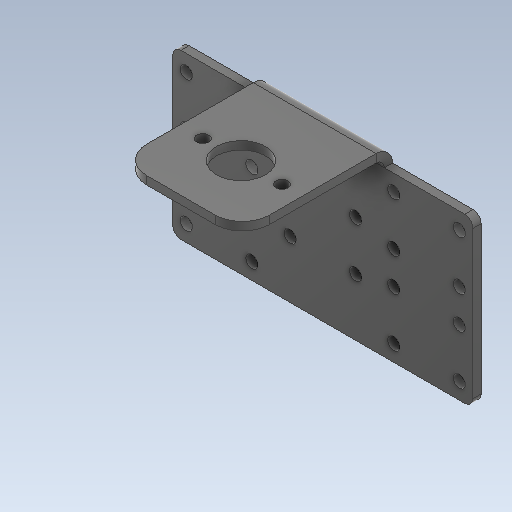
# Autodesk Inventor part: De truc Z chan sat
Saved by Autodesk Inventor 2020 (Build 240168000, 168)
## iProperties
Created: 2021-05-25
Part Number: De truc Z chan sat
Material: Generic
Document SubType Name: Sheet Metal
Designer: admin
Density: 1 g/cm^3
Sheet Metal Rule: Default_mm
Appearance: Smooth - Black
Author: admin
Autodesk Inventor part; units mm, degrees
ref_plane "YZ Plane" through (0, 0, 0) normal (1, 0, 0) x (0, 1, 0)
ref_plane "XZ Plane" through (0, 0, 0) normal (0, 1, 0) x (-1, 0, 0)
ref_plane "XY Plane" through (0, 0, 0) normal (0, 0, 1) x (1, 0, 0)
sketch "Sketch1" plane through (0, 0, 0) normal (0, 0, 1) x (1, 0, 0)
  line L0 (-55, -30) -> (55, -30)
  line L1 (55, -30) -> (55, 30)
  line L2 (55, 30) -> (-55, 30)
  line L3 (-55, 30) -> (-55, -30)
  line L4 (-55, -30) -> (55, 30) construction
  line L5 (55, -30) -> (-55, 30) construction
  line L6 (0, -42) -> (0, 42)
  point P0 (0, 0)
  dimension "d1" = 110
  dimension "d2" = 60
  dimension "d60" = 0
  measures "d1" distance of L2.end L1.end
  measures "d2" distance of L1.end L0.end
  measures "d60" distance from line of point (0, 0) L6
extrude "Plate1" add sketch "Sketch1" along normal blind 3
sketch "Sketch2" plane through (0, 0, 3) normal (0, 0, 1) x (1, 0, 0)
  line L0 (26, -24) -> (50, -24)
  line L1 (50, -24) -> (50, -6)
  line L2 (50, -6) -> (26, -6)
  line L3 (26, -6) -> (26, -24)
  line L4 (26, -24) -> (50, -6) construction
  line L5 (50, -24) -> (26, -6) construction
  circle A0 centre (50, -6) radius 2.25
  circle A1 centre (50, -24) radius 2.25
  circle A2 centre (26, -24) radius 2.25
  circle A3 centre (26, -6) radius 2.25
  line L6 (55, 30) -> (55, -30) projected
  line L7 (55, -30) -> (-55, -30) projected
  point P0 (0, 0)
  point P1 (0, 0)
  point P2 (38, -15)
  dimension "d4" = 24
  dimension "d5" = 18
  dimension "d8" = 4.5
  dimension "d9" = 4.5
  dimension "d10" = 4.5
  dimension "d11" = 4.5
  dimension "d12" = 5
  dimension "d13" = 15
  constraints: 12 end point, 4 centre point, 4 coincident, 2 midpoint, 2 parallel, 1 horizontal, 1 perpendicular
  measures "d4" distance of L2.end L1.end
  measures "d5" distance of L1.end L1.start
  measures "d8" diameter of A0
  measures "d9" diameter of A1
  measures "d10" diameter of A2
  measures "d11" diameter of A3
  measures "d12" distance between parallel lines of L6 L1
  measures "d13" distance from line of L7 point (38, -15)
extrude "Cut1" cut sketch "Sketch2" against normal blind 3 contours L3 A2 L0 | L0 A2 L3 | A1 L1 L0 | L0 L1 A1 | A3 L2 L3 | L3 L2 A3 | A0 L2 L1 | L1 L2 A0
pattern_linear "Rectangular Pattern1" count 2 spacing 30 along (0, 1, 0) of "Cut1"
mirror "Mirror1" about plane through (0, 0, 0) normal (1, 0, 0) of "Cut1", "Rectangular Pattern1"
sketch "Sketch3" plane through (0, 0, 3) normal (0, 0, 1) x (1, 0, 0)
  line L0 (-12, -9) -> (12, -9)
  line L1 (12, -9) -> (12, 9)
  line L2 (12, 9) -> (-12, 9)
  line L3 (-12, 9) -> (-12, -9)
  line L4 (-12, -9) -> (12, 9) construction
  line L5 (12, -9) -> (-12, 9) construction
  circle A0 centre (-12, 9) radius 2.25
  circle A1 centre (12, 9) radius 2.25
  circle A2 centre (12, -9) radius 2.25
  circle A3 centre (-12, -9) radius 2.25
  line L6 (-77, 0) -> (77, 0) projected
  line L7 (0, -42) -> (0, 42) projected
  point P0 (0, 0)
  dimension "d20" = 24
  dimension "d21" = 18
  dimension "d22" = 4.5
  dimension "d23" = 4.5
  dimension "d24" = 4.5
  dimension "d25" = 4.5
  dimension "d26" = 12
  dimension "d27" = 9
  constraints: 12 end point, 4 centre point, 4 coincident, 2 midpoint, 2 parallel, 1 horizontal, 1 perpendicular
  measures "d20" distance of L2.end L1.end
  measures "d21" distance of L1.end L0.end
  measures "d22" diameter of A0
  measures "d23" diameter of A1
  measures "d24" diameter of A2
  measures "d25" diameter of A3
  measures "d26" distance between parallel lines of L7 L1
  measures "d27" distance between parallel lines of L6 L2
extrude "Cut2" cut sketch "Sketch3" against normal blind 3 contours L3 A3 L0 | L0 A3 L3 | A2 L1 L0 | L0 L1 A2 | A0 L2 L3 | L3 L2 A0 | A1 L2 L1 | L1 L2 A1
sketch "Sketch4" plane through (0, 0, 3) normal (0, 0, 1) x (1, 0, 0)
  line L0 (-55, 30) -> (55, 30)
  line L1 (-22.5, 30) -> (22.5, 30)
  line L2 (22.5, 30) -> (22.5, 33)
  line L3 (22.5, 33) -> (-22.5, 33)
  line L4 (-22.5, 33) -> (-22.5, 30)
  point P0 (0, 0)
  point P1 (-50, 30)
  point P2 (50, 30)
  dimension "d30" = 45
  dimension "d31" = 3
  dimension "d32" = 22.5
  measures "d30" distance of L3.end L2.end
  measures "d31" distance of L2.end L1.end
  measures "d32" distance from line of L4 point (0, 0)
sheet face with bend "Face2" sketch "Sketch4" thickness 3 toward (0, 0, -1) bend radius 3
bend "Bend1"
sketch "Sketch5" plane through (-22.5, 33, 3) normal (0, 1, 0) x (-1, 0, 0)
  line L0 (-45, 0) -> (0, 0)
  line L1 (0, 0) -> (0, 52)
  line L2 (0, 52) -> (-45, 52)
  line L3 (-45, 52) -> (-45, 0)
  constraints: 6 end point, 1 horizontal, 1 perpendicular, 1 vertical
edge flange "Flange1" height 55 angle 90 thickness 3 bend radius 3 thickness toward (0, 1, 0) relief tear relief width 3 relief depth 1.5 edges at (0, 33, 3) wall of the first edge with corners at (22.5, 33, 3) (-22.5, 33, 3) (-22.5, 33, 55) (22.5, 33, 55)
bend "Bend2"
corner "Corner1"
sketch "Sketch6" plane through (-22.5, 36, 55) normal (0, 1, 0) x (1, 0, 0)
  circle A0 centre (22.5, 22) radius 9
  line L0 (0, 55) -> (45, 55) projected
  circle A1 centre (37.5, 22) radius 2.25
  circle A2 centre (8.5, 22) radius 2.25
  line L1 (45, 49) -> (45, 0) projected
  line L2 (45, 55) -> (0, 55) projected
  point P0 (22.5, 55)
  point P1 (-25, 55)
  dimension "d48" = 18
  dimension "d49" = 33
  dimension "d50" = 4.5
  dimension "d51" = 4.5
  dimension "d52" = 29
  dimension "d53" = 22.5
  dimension "d54" = 15
  dimension "d55" = 33
  dimension "d56" = 33
  constraints: 3 centre point
  measures "d48" diameter of A0
  measures "d49" distance from line of L0 A0.centre
  measures "d50" diameter of A1
  measures "d51" diameter of A2
  measures "d52" distance of A2.centre A1.centre
  measures "d53" distance from line of L1 A0.centre
  measures "d54" distance of A1.centre A0.centre
  measures "d55" distance from line of L2 A1.centre
  measures "d56" distance from line of L2 A2.centre
extrude "Cut3" cut sketch "Sketch6" against normal blind 3
fillet "Fillet2" radius 10 2 edges at (22.5, 34.5, 55) (-22.5, 34.5, 55)
fillet "Fillet4" radius 3 4 edges at (55, 30, 1.5) (55, -30, 1.5) (-55, -30, 1.5) (-55, 30, 1.5)
equation "\"d14\" = Thickness"
equation "\"d28\" = Thickness"
equation "\"d57\" = Thickness"
equation "\"d3\" = Thickness"
equation "\"d33\" = BendRadius"
equation "\"d34\" = BendReliefWidth"
equation "\"d36\" = MinimumRemnant"
equation "\"d35\" = BendReliefDepth"
equation "\"d37\" = TransitionRadius"
equation "\"d38\" = BendReliefWidth"
equation "\"d39\" = BendReliefDepth"
equation "\"d40\" = MinimumRemnant"
equation "\"d41\" = TransitionRadius"
equation "\"d44\" = BendRadius"
equation "\"d45\" = CornerReliefSize"
equation "\"d46\" = GapSize"
equation "\"d47\" = JacobiRadiusSize"
equation "\"BendRadius\" = Thickness"
equation "\"BendReliefWidth\" = Thickness"
equation "\"BendReliefDepth\" = 0.5 * Thickness"
equation "\"CornerReliefSize\" = 4 * Thickness"
equation "\"MinimumRemnant\" = 2 * Thickness"
equation "\"TransitionRadius\" = BendRadius"
equation "\"JacobiRadiusSize\" = BendRadius"
equation "\"GapSize\" = Thickness"
equation "\"Thickness\" = 3"
body "Solid1"
